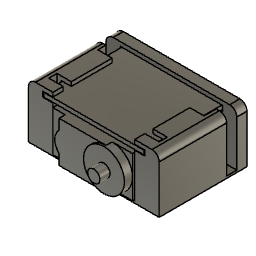
rest v6 (Autodesk Fusion 360 design; units mm, degrees)
Autodesk Fusion 360 part; units mm, degrees
note: some values were not read from the file. Set by a fixed rule: which sketch regions a step uses.
sketch "Sketch1" plane through (0, 0, 0) normal (0, 1, 0) x (1, 0, 0) in component "actual acutator v0 v1"
  line L0 (0, 0) -> (53, 0)
  line L1 (53, 0) -> (53, -39)
  line L2 (53, -39) -> (0, -39)
  line L3 (0, -39) -> (0, 0)
  dimension "d1" = 53
  dimension "d2" = 39
  constraint horizontal L0
  constraint vertical L1
  constraint horizontal L2
  constraint vertical L3
  constraint coincident L0.start L3.end
  measures "d1" distance of L0.start L0.end
  measures "d2" distance of L0.start L2.end
extrude "Extrude1" add sketch "Sketch1" along normal blind 20 makes body 1 in component "actual acutator v0 v1"
sketch "Sketch2" plane through (0, 0, 39) normal (0, 0, 1) x (-1, 0, 0) in component "actual acutator v0 v1"
  line L0 (0, 0) -> (-53, 0)
  line L1 (-53, 0) -> (-53, -20)
  line L2 (-53, -20) -> (0, -20)
  line L3 (0, -20) -> (0, 0)
  line L4 (0, -20) -> (-7, -20)
  line L5 (-7, -20) -> (-7, 0)
  line L6 (-7, 0) -> (0, 0)
  line L7 (0, 0) -> (0, -20)
  line L8 (-53, -20) -> (-46, -20)
  line L9 (-46, -20) -> (-46, 0)
  line L10 (-46, 0) -> (-53, 0)
  line L11 (-53, 0) -> (-53, -20)
  dimension "d5" = 7
  dimension "d6" = 7
  constraint horizontal L4
  constraint vertical L5
  constraint horizontal L6
  constraint vertical L7
  constraint coincident L2.end L3.start
  constraint horizontal L8
  constraint vertical L9
  constraint horizontal L10
  constraint vertical L11
  constraint coincident L0 L9.end
  constraint coincident L1.end L2.start
  measures "d5" distance of L2.end L4.end
  measures "d6" distance of L1.end L8.end
extrude "Extrude2" cut sketch "Sketch2" against normal blind 10 contours L0 L2 L3 L4 L5 L6 L7 | L0 L1 L2 L8 L9 L10 L11 bodies 1 in component "actual acutator v0 v1"
sketch "Sketch3" plane through (0, 0, 0) normal (0, 0, -1) x (1, 0, 0) in component "actual acutator v0 v1"
  line L0 (53, 0) -> (0, 0)
  line L1 (0, 0) -> (0, -20)
  line L2 (0, -20) -> (53, -20)
  line L3 (53, -20) -> (53, 0)
  line L4 (0, 0) -> (7, 0)
  line L5 (7, 0) -> (7, -20)
  line L6 (7, -20) -> (0, -20)
  line L7 (0, -20) -> (0, 0)
  line L8 (53, 0) -> (46, 0)
  line L9 (46, 0) -> (46, -20)
  line L10 (46, -20) -> (53, -20)
  line L11 (53, -20) -> (53, 0)
  dimension "d9" = 7
  dimension "d10" = 7
  constraint horizontal L4
  constraint vertical L5
  constraint horizontal L6
  constraint vertical L7
  constraint coincident L0.end L1.start
  constraint horizontal L8
  constraint vertical L9
  constraint horizontal L10
  constraint vertical L11
  constraint coincident L0.start L3.end
  measures "d9" distance of L0.end L4.end
  measures "d10" distance of L0.start L8.end
extrude "Extrude3" cut sketch "Sketch3" against normal blind 26 contours L0 L2 L3 L8 L9 L10 L11 | L0 L1 L2 L4 L5 L6 L7 bodies 1 in component "actual acutator v0 v1"
sketch "Sketch4" plane through (0, 0, 39) normal (0, 0, 1) x (-1, 0, 0) in component "actual acutator v0 v1"
  line L0 (-7, -20) -> (-7, 0)
  line L1 (-7, 0) -> (-46, 0)
  line L2 (-46, 0) -> (-46, -20)
  line L3 (-46, -20) -> (-7, -20)
  line L4 (-7, -20) -> (-13, -20)
  line L5 (-13, -20) -> (-13, 0)
  line L6 (-13, 0) -> (-7, 0)
  line L7 (-7, 0) -> (-7, -20)
  circle A0 centre (-36, -10) radius 10
  circle A1 centre (-36, -10) radius 6.5
  circle A2 centre (-36, -10) radius 3
  spline S0 degree 5 poles (-13, -15.0203) (-12.838, -14.8194) (-12.5281, -14.4176) (-12.1057, -13.8151) (-11.6287, -13.012) (-11.1861, -12.0086) (-10.9107, -11.0057) (-10.8163, -10.0034) (-10.9104, -9.0017) (-11.1856, -8.0005) (-11.6282, -6.9998) (-12.1053, -6.1997) (-12.5279, -5.5998) (-12.8379, -5.1999) (-13, -5) knots 0 0 0 0 0 0 0.1 0.2 0.3 0.4 0.5 0.6 0.7 0.8 0.9 1 1 1 1 1 1
  point P0 (-13, -10)
  point P1 (-13, -15.0203)
  point P2 (-13, -5)
  point P3 (-10.8633, -10)
  dimension "d13" = 6
  dimension "d14" = 20
  dimension "d15" = 13
  dimension "d16" = 6
  constraint horizontal L4
  constraint vertical L5
  constraint horizontal L6
  constraint vertical L7
  constraint coincident L0.start L3.end
  constraint tangent L3 A0
  constraint tangent L2 A0
  constraint tangent L1 A0
  constraint concentric A0 A1
  constraint concentric A1 A2
  constraint midpoint L5 P0
  constraint coincident L5 P1
  constraint coincident L5 P2
  constraint coincident P2 S0.end
  measures "d13" distance of L0.start L4.end
  measures "d14" distance of L0.start L0.end
  measures "d15" diameter of A1
  measures "d16" diameter of A2
extrude "Extrude4" cut sketch "Sketch4" against normal blind 4 contours L0 L1 L3 L4 L5 L6 L7 S0 | L2 L3 A0 | L1 L2 A0 bodies 1 in component "actual acutator v0 v1"
extrude "Extrude5" cut sketch "Sketch4" against normal blind 1 contours L1 L3 L5 A0 | L2 L3 A0 | L5 S0 | L1 L2 A0 bodies 1 in component "actual acutator v0 v1"
extrude "Extrude6" add sketch "Sketch4" along normal blind 5 contours A2 bodies 1 in component "actual acutator v0 v1"
sketch "Sketch5" plane through (0, 0, 29) normal (0, 0, 1) x (-1, 0, 0) in component "actual acutator v0 v1"
  line L0 (-53, 0) -> (-53, -20)
  line L1 (-53, -20) -> (-46, -20)
  line L2 (-46, -20) -> (-46, 0)
  line L3 (-46, 0) -> (-53, 0)
  line L4 (-53, 0) -> (-51, 0)
  line L5 (-51, 0) -> (-51, -5)
  line L6 (-51, -5) -> (-53, -5)
  line L7 (-53, -5) -> (-53, 0)
  circle A0 centre (-51, -5) radius 2
  line L8 (-53, -20) -> (-51, -20)
  line L9 (-51, -20) -> (-51, -15)
  line L10 (-51, -15) -> (-53, -15)
  line L11 (-53, -15) -> (-53, -20)
  circle A1 centre (-51, -15) radius 2
  dimension "d23" = 2
  dimension "d24" = 5
  dimension "d25" = 4
  dimension "d26" = 2
  dimension "d27" = 5
  dimension "d28" = 4
  constraint horizontal L4
  constraint vertical L5
  constraint horizontal L6
  constraint vertical L7
  constraint coincident L0.start L3.end
  constraint coincident L5.end L6.start
  constraint horizontal L8
  constraint vertical L9
  constraint horizontal L10
  constraint vertical L11
  constraint coincident L0.end L1.start
  constraint coincident L9.end L10.start
  measures "d23" distance of L0.start L4.end
  measures "d24" distance of L0.start L6.end
  measures "d25" diameter of A0
  measures "d26" distance of L0.end L8.end
  measures "d27" distance of L0.end L10.end
  measures "d28" diameter of A1
extrude "Extrude7" cut sketch "Sketch5" against normal blind 3 contours L5 L6 A0 | L5 L6 A0 | L9 L10 A1 | L9 L10 A1 bodies 1 in component "actual acutator v0 v1"
ref_plane "WorkPlane1" through (26.5, 0, 0) normal (1, 0, 0) x (0, 1, 0) in component "actual acutator v0 v1"
mirror "Mirror1" about plane through (26.5, 0, 0) normal (1, 0, 0) of "Extrude7" in component "actual acutator v0 v1"
sketch "Sketch1 (2)" plane through (0, 0, 0) normal (0, 0, 1) x (1, 0, 0) in component "casing"
  line L0 (-13.5, -7.7959) -> (9.5, -7.7959)
  line L1 (9.5, -7.7959) -> (9.5, -4.7959)
  line L2 (9.5, -4.7959) -> (19.5, -4.7959)
  line L3 (19.5, -4.7959) -> (19.5, 1.2041)
  line L4 (19.5, 1.2041) -> (26.5, 1.2041)
  line L5 (26.5, 1.2041) -> (26.5, 4.2041)
  line L6 (26.5, 4.2041) -> (19.5, 4.2041)
  line L7 (19.5, 4.2041) -> (19.5, 30.2041)
  line L8 (19.5, 30.2041) -> (-19.5, 30.2041)
  line L9 (-19.5, 30.2041) -> (-19.5, 4.2041)
  line L10 (-19.5, 4.2041) -> (-26.5, 4.2041)
  line L11 (-26.5, 4.2041) -> (-26.5, 1.2041)
  line L12 (-26.5, 1.2041) -> (-19.5, 1.2041)
  line L13 (-19.5, 1.2041) -> (-19.5, -4.7959)
  line L14 (-19.5, -4.7959) -> (-13.5, -4.7959)
  line L15 (-13.5, -4.7959) -> (-13.5, -7.7959)
  line L16 (-20, 0.7041) -> (-32, 0.7041)
  line L17 (-32, 0.7041) -> (-32, -4.2959)
  line L18 (-32, -4.2959) -> (-20, -4.2959)
  line L19 (-20, -4.2959) -> (-20, 0.7041)
  line L20 (-32, 0.7041) -> (-27, 0.7041)
  line L21 (-27, 0.7041) -> (-27, 38.7041)
  line L22 (-27, 38.7041) -> (-32, 38.7041)
  line L23 (-32, 38.7041) -> (-32, 0.7041)
  line L24 (-27, 38.7041) -> (27, 38.7041)
  line L25 (27, 38.7041) -> (27, 33.7041)
  line L26 (27, 33.7041) -> (-27, 33.7041)
  line L27 (-27, 33.7041) -> (-27, 38.7041)
  line L28 (20, 0.7041) -> (32, 0.7041)
  line L29 (32, 0.7041) -> (32, -4.2959)
  line L30 (32, -4.2959) -> (20, -4.2959)
  line L31 (20, -4.2959) -> (20, 0.7041)
  line L32 (32, 0.7041) -> (27, 0.7041)
  line L33 (27, 0.7041) -> (27, 38.7041)
  line L34 (27, 38.7041) -> (32, 38.7041)
  line L35 (32, 38.7041) -> (32, 0.7041)
  line L36 (27, 4.7041) -> (20, 4.7041)
  line L37 (20, 4.7041) -> (20, 22.7041)
  line L38 (20, 22.7041) -> (27, 22.7041)
  line L39 (27, 22.7041) -> (27, 4.7041)
  line L40 (-27, 4.7041) -> (-20, 4.7041)
  line L41 (-20, 4.7041) -> (-20, 24.7041)
  line L42 (-20, 24.7041) -> (-27, 24.7041)
  line L43 (-27, 24.7041) -> (-27, 4.7041)
  line L44 (-32, 38.7041) -> (32, 38.7041)
  line L45 (32, 38.7041) -> (32, -4.2959)
  line L46 (32, -4.2959) -> (-32, -4.2959)
  line L47 (-32, -4.2959) -> (-32, 38.7041)
  line L48 (-27, 33.7041) -> (-32, 33.7041)
  line L49 (-32, 33.7041) -> (-32, 28.7041)
  line L50 (-32, 28.7041) -> (-27, 28.7041)
  line L51 (-27, 28.7041) -> (-27, 33.7041)
  line L52 (27, 33.7041) -> (32, 33.7041)
  line L53 (32, 33.7041) -> (32, 28.7041)
  line L54 (32, 28.7041) -> (27, 28.7041)
  line L55 (27, 28.7041) -> (27, 33.7041)
  dimension "d34" = 0.5
  dimension "d35" = 0.5
  dimension "d36" = 5
  dimension "d37" = 12
  dimension "d38" = 0.5
  dimension "d39" = 3.5
  dimension "d40" = 5
  dimension "d41" = 0.5
  dimension "d42" = 0.5
  dimension "d43" = 12
  dimension "d44" = 5
  dimension "d45" = 0.5
  dimension "d46" = 0.5
  dimension "d47" = 0.5
  dimension "d48" = 18
  dimension "d49" = 0.5
  dimension "d50" = 0.5
  dimension "d51" = 20
  dimension "d56" = 5
  dimension "d57" = 5
  constraint horizontal L16
  constraint vertical L17
  constraint horizontal L18
  constraint vertical L19
  constraint horizontal L20
  constraint vertical L21
  constraint horizontal L22
  constraint vertical L23
  constraint horizontal L24
  constraint vertical L25
  constraint horizontal L26
  constraint vertical L27
  constraint horizontal L28
  constraint vertical L29
  constraint horizontal L30
  constraint vertical L31
  constraint horizontal L32
  constraint vertical L33
  constraint horizontal L34
  constraint vertical L35
  constraint horizontal L36
  constraint vertical L37
  constraint horizontal L38
  constraint vertical L39
  constraint coincident L33 L36.start
  constraint horizontal L40
  constraint vertical L41
  constraint horizontal L42
  constraint vertical L43
  constraint coincident L21 L40.start
  constraint horizontal L44
  constraint vertical L45
  constraint horizontal L46
  constraint vertical L47
  constraint horizontal L48
  constraint vertical L49
  constraint horizontal L50
  constraint vertical L51
  constraint coincident L47 L49.end
  constraint horizontal L52
  constraint vertical L53
  constraint horizontal L54
  constraint vertical L55
  constraint coincident L45 L53.end
  measures "d34" distance of L13 L19
  measures "d35" distance of L12 L16
  measures "d36" distance of L16.end L17.end
  measures "d37" distance of L17.end L18.end
  measures "d38" distance of L11 L21
  measures "d39" distance of L8 L26
  measures "d40" distance of L24.end L25.end
  measures "d41" distance of L4 L28
  measures "d42" distance of L3 L31
  measures "d43" distance of L29.end L30.end
  measures "d44" distance of L28.end L29.end
  measures "d45" distance of L5 L33
  measures "d46" distance of L6 L36
  measures "d47" distance of L7 L37
  measures "d48" distance of L36.end L37.end
  measures "d49" distance of L10 L40
  measures "d50" distance of L9 L41
  measures "d51" distance of L40 L42
  measures "d56" distance of L48 L50
  measures "d57" distance of L52 L54
extrude "Extrude1'" add sketch "Sketch1 (2)" against normal blind 1 separate body contours L3 L4 L5 L6 L7 L8 L9 L10 L11 L12 L13 L16 L19 L21 L26 L28 L31 L33 L36 L37 L38 L40 L41 L42 L46 L51 L55 | L3 L4 L5 L6 L7 L8 L9 L10 L11 L12 L13 L46 | L16 L17 L18 L19 L20 L46 L47 | L28 L29 L30 L31 L32 L45 L46 | L16 L20 L21 L23 L43 L47 L50 | L28 L32 L33 L35 L39 L45 L54 | L21 L23 L47 L48 L49 L50 L51 | L21 L40 L41 L42 L43 | L33 L35 L45 L52 L53 L54 L55 | L33 L36 L37 L38 L39 | L21 L22 L23 L27 L44 L47 L48 | L25 L33 L34 L35 L44 L45 L52 | L21 L24 L25 L26 L27 L33 L44 makes body 2 in component "casing"
extrude "Extrude2'" add sketch "Sketch1 (2)" along normal blind 26 contours L16 L17 L18 L19 L20 L46 L47 | L28 L29 L30 L31 L32 L45 L46 | L16 L20 L21 L23 L43 L47 L50 | L28 L32 L33 L35 L39 L45 L54 | L21 L40 L41 L42 L43 | L33 L36 L37 L38 L39 | L21 L22 L23 L27 L44 L47 L48 | L25 L33 L34 L35 L44 L45 L52 | L21 L24 L25 L26 L27 L33 L44 bodies 2 in component "casing"
sketch "Sketch2 (2)" plane through (0, -4.2959, 0) normal (0, -1, 0) x (1, 0, 0) in component "casing"
  line L0 (20, 0) -> (-20, 0)
  line L1 (-20, 0) -> (-20, 26)
  line L2 (-20, 26) -> (-32, 26)
  line L3 (-32, 26) -> (-32, -1)
  line L4 (-32, -1) -> (32, -1)
  line L5 (32, -1) -> (32, 26)
  line L6 (32, 26) -> (20, 26)
  line L7 (20, 26) -> (20, 0)
  line L8 (-25, 24) -> (25, 24)
  line L9 (25, 24) -> (25, 21.5)
  line L10 (25, 21.5) -> (-25, 21.5)
  line L11 (-25, 21.5) -> (-25, 24)
  line L12 (-32, 26) -> (32, 26)
  dimension "d58" = 2.5
  dimension "d59" = 50
  dimension "d60" = 2
  dimension "d61" = 7
  constraint horizontal L8
  constraint vertical L9
  constraint horizontal L10
  constraint vertical L11
  measures "d58" distance of L8.start L10.end
  measures "d59" distance of L8.start L8.end
  measures "d60" distance of L8 L12
  measures "d61" distance of L5 L9
extrude "Extrude3'" cut sketch "Sketch2 (2)" against normal blind 40 contours L1 L7 L8 L10 | L7 L8 L9 L10 | L1 L8 L10 L11 bodies 2 in component "casing"
sketch "Sketch1 (3)" plane through (0, -4.2959, 0) normal (0, -1, 0) x (1, 0, 0) in component "lid"
  line L0 (-20, 21.5) -> (-25, 21.5)
  line L1 (-25, 21.5) -> (-25, 24)
  line L2 (-25, 24) -> (-20, 24)
  line L3 (-20, 24) -> (-20, 26)
  line L4 (-20, 26) -> (-32, 26)
  line L5 (-32, 26) -> (-32, -1)
  line L6 (-32, -1) -> (32, -1)
  line L7 (32, -1) -> (32, 26)
  line L8 (32, 26) -> (20, 26)
  line L9 (20, 26) -> (20, 24)
  line L10 (20, 24) -> (25, 24)
  line L11 (25, 24) -> (25, 21.5)
  line L12 (25, 21.5) -> (20, 21.5)
  line L13 (20, 21.5) -> (20, 0)
  line L14 (20, 0) -> (-20, 0)
  line L15 (-20, 0) -> (-20, 21.5)
  line L16 (24.5, 21.75) -> (-24.5, 21.75)
  line L17 (-24.5, 21.75) -> (-24.5, 23.75)
  line L18 (-24.5, 23.75) -> (24.5, 23.75)
  line L19 (24.5, 23.75) -> (24.5, 21.75)
  line L20 (24.5, 21.75) -> (-24.5, 23.75) construction
  line L21 (-24.5, 21.75) -> (24.5, 23.75) construction
  point P0 (0, 22.75)
  dimension "d64" = 49
  dimension "d65" = 2
  dimension "d66" = 2.25
  dimension "d67" = 0.5
  constraint horizontal L16
  constraint perpendicular L16 L17
  constraint parallel L16 L18
  constraint parallel L17 L19
  constraint coincident L20 P0
  constraint coincident L21 P0
  measures "d64" distance of L17.end L18.end
  measures "d65" distance of L16.end L17.end
  measures "d66" distance of L8 L18
  measures "d67" distance of L11 L19
extrude "Extrude1''" add sketch "Sketch1 (3)" against normal blind 39 separate body contours L16 L17 L18 L19 makes body 3 in component "lid"
fillet "Fillet1" radius 3.5 4 edges at (-32, 12.2041, 26) (32, 12.2041, 26) (32, 36.2041, 26) (-32, 36.2041, 26) on bodies 2 in component "casing"
component "actual acutator v0 v1" placed x (1, 0, 0) y (0, 0, 1) z (0, -1, 0) at (-26.5, 30.2041, 0.0041)
component "casing" placed x (1, 0, 0) y (0, 1, 0) z (0, 0, 1) at (0, 0, 0)
component "lid" placed x (1, 0, 0) y (0, 1, 0) z (0, 0, 1) at (0, 0, 0) in component "casing"
